Autodesk Inventor part; units mm, degrees
(part 2 of 3)
extrude "Extrusion14" add sketch "Sketch20" against normal blind 2.54 contours L123 L124 L125 L126 L127 L128 L129 L130 L131 L132 L133 L134 | L151 L152 L153 L154 L155 L156 | L181 L182 L183 L184 L185 L186 | L204 L197 L198 L199 L200 L201 L202 L203 | S194 S179 A0 | A0 S179 S180 S181 S182 S183 S184 L205 L206 S185 S186 S187 S188 S189 S190 S191 S192 L207 L208 S193 S194 | S73 S74 S75 S76 S77 S78 L135 L136 S79 S80 S81 S82 S83 S84 S85 S86 L137 L138 S87 S88 A0 | A0 S88 S73 | S92 S93 S94 S95 S96 S89 S90 S91 A0 | A0 S91 S92 | S167 S168 A0 | A0 S168 S169 S170 S171 S172 S165 S166 S167 | S153 S154 A0 | A0 S154 S155 S156 S157 S158 S151 S152 S153 | S103 L157 L158 S104 S105 S106 S107 S108 S109 S110 S111 L159 L160 S112 S113 S114 S115 S116 S117 S118 A0 | A0 S118 S103 | S150 S135 A0 | A0 S135 S136 S137 S138 S139 S140 L165 L166 S141 S142 S143 S144 S145 S146 S147 S148 L167 L168 S149 S150 | S119 L161 L162 S120 S121 S122 S123 S124 S125 S126 S127 L163 L164 S128 S129 S130 S131 S132 S133 S134 A0 | A0 S134 S119 | S0 S1 L0 L1 L2 L3 L4 S2 S3 | L8 L9 L10 L11 L12 L13 L14 L15 L16 L17 L18 L19 | L20 L21 L22 L23 L24 L25 L26 L27 L28 L29 L30 L31 | L32 L33 L34 L35 L36 L37 L38 S8 S9 S10 L39 | L43 L44 L45 L46 L47 L48 L49 L50 | L54 L55 L56 L57 L58 L59 L60 L61 L62 L63 L64 L65 L66 | L67 L68 L69 L70 L71 L72 L73 L74 | L78 L79 L80 L81 L82 L83 L84 S15 S16 S17 L85 | S22 S23 L89 L90 L91 S24 S25 | L95 L96 S30 S31 S32 S33 S34 S35 L97 L98 S36 S37 S38 S39 S40 L99 L100 | S41 S42 S43 S44 | L101 L102 L103 L104 L105 L106 S53 L107 L108 L109 L110 | S54 S55 S56 L111 S57 S58 S59 S60 L112 S61 S62 | L113 L114 L115 L116 L117 L118 L119 L120 L121 L122 | L139 L140 L141 L142 L143 L144 L145 L146 L147 L148 L149 L150 | L169 L170 L171 L172 L173 L174 L175 L176 L177 L178 L179 L180 | L187 L188 L189 L190 L191 L192 L193 L194 L195 L196
sketch "Sketch21" plane through (27.94, 0, 0) normal (1, 0, 0) x (0, 0, -1)
  point P0 (0, 0)
sketch "Sketch22" plane through (25.4, 0, 0) normal (1, 0, 0) x (0, 0, -1)
  circle A0 centre (0, 0) radius 75.606
  line L0 (-75.2037, 22.4511) -> (-75.7978, 19.48)
  line L1 (-75.7978, 19.48) -> (-94.7412, 14.099)
  line L2 (-94.7412, 14.099) -> (-77.5606, 10.6637)
  line L3 (-77.5606, 10.6637) -> (-78.0546, 8.1932)
  line L4 (-78.0546, 8.1932) -> (-97.9802, 12.1773)
  line L5 (-97.9802, 12.1773) -> (-97.2279, 15.9396)
  line L6 (-97.2279, 15.9396) -> (-79.8475, 20.8104)
  line L7 (-79.8475, 20.8104) -> (-95.6233, 23.9648)
  line L8 (-95.6233, 23.9648) -> (-95.1293, 26.4353)
  line L9 (-95.1293, 26.4353) -> (-75.2037, 22.4511)
  line L10 (-71.0246, 32.8287) -> (-73.9643, 25.5272)
  line L11 (-73.9643, 25.5272) -> (-75.8889, 26.3021)
  line L12 (-75.8889, 26.3021) -> (-74.9234, 28.7003)
  line L13 (-74.9234, 28.7003) -> (-89.9237, 34.7395)
  line L14 (-89.9237, 34.7395) -> (-90.8892, 32.3413)
  line L15 (-90.8892, 32.3413) -> (-92.8139, 33.1162)
  line L16 (-92.8139, 33.1162) -> (-89.8742, 40.4178)
  line L17 (-89.8742, 40.4178) -> (-87.9496, 39.6429)
  line L18 (-87.9496, 39.6429) -> (-88.9151, 37.2447)
  line L19 (-88.9151, 37.2447) -> (-73.9148, 31.2054)
  line L20 (-73.9148, 31.2054) -> (-72.9493, 33.6036)
  line L21 (-72.9493, 33.6036) -> (-71.0246, 32.8287)
  spline S0 degree 2 poles (-65.2074, 42.4368) (-66.2508, 40.7587) (-69.1486, 38.6243) (-70.9248, 38.2938) knots 0 0 0 1 2 2 2
  spline S1 degree 2 poles (-70.9248, 38.2938) (-72.6869, 37.9546) (-76.7474, 38.9088) (-78.9288, 40.2652) knots 0 0 0 1 2 2 2
  spline S2 degree 2 poles (-78.9288, 40.2652) (-81.0963, 41.613) (-83.6257, 44.7176) (-84.1622, 46.5055) knots 0 0 0 1 2 2 2
  spline S3 degree 2 poles (-84.1622, 46.5055) (-84.6794, 48.262) (-84.1396, 51.8432) (-83.0527, 53.5912) knots 0 0 0 1 2 2 2
  spline S4 degree 2 poles (-83.0527, 53.5912) (-82.5136, 54.4582) (-81.3141, 55.8259) (-80.7183, 56.3475) knots 0 0 0 1 2 2 2
  spline S5 degree 2 poles (-80.7183, 56.3475) (-80.1887, 56.7938) (-78.9496, 57.6327) (-78.2855, 58.0148) knots 0 0 0 1 2 2 2
  line L22 (-78.2855, 58.0148) -> (-75.5167, 56.2931)
  line L23 (-75.5167, 56.2931) -> (-75.6297, 56.1113)
  spline S6 degree 2 poles (-75.6297, 56.1113) (-76.1007, 55.9776) (-77.475, 55.5136) (-78.2787, 55.0632) knots 0 0 0 1 2 2 2
  spline S7 degree 2 poles (-78.2787, 55.0632) (-79.0509, 54.632) (-80.4776, 53.3667) (-81.1036, 52.3599) knots 0 0 0 1 2 2 2
  spline S8 degree 2 poles (-81.1036, 52.3599) (-81.7905, 51.2552) (-82.1076, 48.7183) (-81.7015, 47.438) knots 0 0 0 1 2 2 2
  spline S9 degree 2 poles (-81.7015, 47.438) (-81.2726, 46.1631) (-79.106, 43.6912) (-77.442, 42.6565) knots 0 0 0 1 2 2 2
  spline S10 degree 2 poles (-77.442, 42.6565) (-75.666, 41.5522) (-72.5766, 40.814) (-71.2347, 41.0073) knots 0 0 0 1 2 2 2
  spline S11 degree 2 poles (-71.2347, 41.0073) (-69.9296, 41.2041) (-67.8539, 42.6087) (-67.1757, 43.6995) knots 0 0 0 1 2 2 2
  spline S12 degree 2 poles (-67.1757, 43.6995) (-66.5583, 44.6923) (-65.9957, 46.6887) (-65.9506, 47.572) knots 0 0 0 1 2 2 2
  spline S13 degree 2 poles (-65.9506, 47.572) (-65.9229, 48.4274) (-66.0954, 49.8338) (-66.1959, 50.2647) knots 0 0 0 1 2 2 2
  line L24 (-66.1959, 50.2647) -> (-66.0916, 50.4325)
  line L25 (-66.0916, 50.4325) -> (-63.3507, 48.7283)
  spline S14 degree 2 poles (-63.3507, 48.7283) (-63.4415, 47.9897) (-63.5782, 46.6786) (-63.7979, 45.8263) knots 0 0 0 1 2 2 2
  spline S15 degree 2 poles (-63.7979, 45.8263) (-64.0157, 44.9146) (-64.5639, 43.4716) (-65.2074, 42.4368) knots 0 0 0 1 2 2 2
  line L26 (-50.1614, 60.3743) -> (-52.0671, 58.4609)
  line L27 (-52.0671, 58.4609) -> (-59.114, 65.4797)
  line L28 (-59.114, 65.4797) -> (-65.7144, 58.8529)
  line L29 (-65.7144, 58.8529) -> (-58.6676, 51.8341)
  line L30 (-58.6676, 51.8341) -> (-60.5734, 49.9207)
  line L31 (-60.5734, 49.9207) -> (-74.9704, 64.2605)
  line L32 (-74.9704, 64.2605) -> (-73.0646, 66.1739)
  line L33 (-73.0646, 66.1739) -> (-67.4178, 60.5495)
  line L34 (-67.4178, 60.5495) -> (-60.8173, 67.1763)
  line L35 (-60.8173, 67.1763) -> (-66.4641, 72.8007)
  line L36 (-66.4641, 72.8007) -> (-64.5583, 74.7141)
  line L37 (-64.5583, 74.7141) -> (-50.1614, 60.3743)
  spline S16 degree 2 poles (-43.9337, 85.7693) (-42.2501, 85.2061) (-39.1129, 82.481) (-37.8061, 80.3077) knots 0 0 0 1 2 2 2
  spline S17 degree 2 poles (-37.8061, 80.3077) (-36.5333, 78.1909) (-35.5439, 74.1168) (-35.8642, 72.3486) knots 0 0 0 1 2 2 2
  spline S18 degree 2 poles (-35.8642, 72.3486) (-36.2069, 70.4901) (-38.3477, 67.6273) (-40.0553, 66.6006) knots 0 0 0 1 2 2 2
  spline S19 degree 2 poles (-40.0553, 66.6006) (-41.8193, 65.5399) (-45.363, 65.0424) (-47.0974, 65.5943) knots 0 0 0 1 2 2 2
  spline S20 degree 2 poles (-47.0974, 65.5943) (-48.7952, 66.149) (-51.9127, 68.9052) (-53.2025, 71.0502) knots 0 0 0 1 2 2 2
  spline S21 degree 2 poles (-53.2025, 71.0502) (-54.5177, 73.2376) (-55.4336, 77.2214) (-55.1529, 79.0234) knots 0 0 0 1 2 2 2
  spline S22 degree 2 poles (-55.1529, 79.0234) (-54.8326, 80.7916) (-52.7174, 83.6967) (-50.9674, 84.7488) knots 0 0 0 1 2 2 2
  spline S23 degree 2 poles (-50.9674, 84.7488) (-49.1893, 85.818) (-45.5919, 86.2902) (-43.9337, 85.7693) knots 0 0 0 1 2 2 2
  spline S24 degree 2 poles (-40.2193, 78.8567) (-41.2545, 80.5784) (-43.6062, 82.7959) (-44.8097, 83.2636) knots 0 0 0 1 2 2 2
  spline S25 degree 2 poles (-44.8097, 83.2636) (-46.0442, 83.751) (-48.5348, 83.4831) (-49.7484, 82.7534) knots 0 0 0 1 2 2 2
  spline S26 degree 2 poles (-49.7484, 82.7534) (-51.0044, 81.9982) (-52.3693, 79.9862) (-52.529, 78.6221) knots 0 0 0 1 2 2 2
  spline S27 degree 2 poles (-52.529, 78.6221) (-52.6859, 77.3172) (-51.8075, 74.1947) (-50.7893, 72.5012) knots 0 0 0 1 2 2 2
  spline S28 degree 2 poles (-50.7893, 72.5012) (-48.7274, 69.0719) (-43.6593, 67.162) (-41.2461, 68.613) knots 0 0 0 1 2 2 2
  spline S29 degree 2 poles (-41.2461, 68.613) (-38.8329, 70.064) (-38.1573, 75.4275) (-40.2193, 78.8567) knots 0 0 0 1 2 2 2
  line L38 (-18.5674, 76.2196) -> (-29.718, 72.44)
  line L39 (-29.718, 72.44) -> (-36.2411, 91.6845)
  line L40 (-36.2411, 91.6845) -> (-33.6835, 92.5515)
  line L41 (-33.6835, 92.5515) -> (-27.9322, 75.5838)
  line L42 (-27.9322, 75.5838) -> (-19.3392, 78.4965)
  line L43 (-19.3392, 78.4965) -> (-18.5674, 76.2196)
  spline S30 degree 2 poles (-10.8247, 77.0268) (-13.01, 76.7214) (-16.2036, 77.2061) (-17.6484, 77.6692) knots 0 0 0 1 2 2 2
  line L44 (-17.6484, 77.6692) -> (-18.118, 81.0287)
  line L45 (-18.118, 81.0287) -> (-17.9223, 81.0561)
  spline S31 degree 2 poles (-17.9223, 81.0561) (-16.4281, 80.0013) (-12.8934, 79.0987) (-11.3441, 79.3153) knots 0 0 0 1 2 2 2
  spline S32 degree 2 poles (-11.3441, 79.3153) (-9.1262, 79.6253) (-7.1169, 81.785) (-7.3289, 83.3016) knots 0 0 0 1 2 2 2
  spline S33 degree 2 poles (-7.3289, 83.3016) (-7.4976, 84.5084) (-8.8978, 85.8424) (-10.2386, 86.0374) knots 0 0 0 1 2 2 2
  spline S34 degree 2 poles (-10.2386, 86.0374) (-11.2046, 86.1684) (-12.8041, 86.3106) (-14.003, 86.4423) knots 0 0 0 1 2 2 2
  spline S35 degree 2 poles (-14.003, 86.4423) (-15.0855, 86.5737) (-16.8489, 87.1752) (-17.5783, 87.7549) knots 0 0 0 1 2 2 2
  spline S36 degree 2 poles (-17.5783, 87.7549) (-18.2915, 88.3369) (-19.2272, 90.0351) (-19.3913, 91.2093) knots 0 0 0 1 2 2 2
  spline S37 degree 2 poles (-19.3913, 91.2093) (-19.7332, 93.6555) (-16.3799, 97.4995) (-13.4281, 97.9121) knots 0 0 0 1 2 2 2
  spline S38 degree 2 poles (-13.4281, 97.9121) (-11.732, 98.1492) (-8.6378, 97.8999) (-7.2606, 97.444) knots 0 0 0 1 2 2 2
  line L46 (-7.2606, 97.444) -> (-6.8138, 94.2476)
  line L47 (-6.8138, 94.2476) -> (-7.0095, 94.2202)
  spline S39 degree 2 poles (-7.0095, 94.2202) (-8.0948, 94.9664) (-11.2779, 95.8516) (-12.925, 95.6214) knots 0 0 0 1 2 2 2
  spline S40 degree 2 poles (-12.925, 95.6214) (-14.7841, 95.3615) (-16.8397, 93.2951) (-16.6414, 91.8763) knots 0 0 0 1 2 2 2
  spline S41 degree 2 poles (-16.6414, 91.8763) (-16.4636, 90.6043) (-14.898, 89.2768) (-13.5781, 89.1121) knots 0 0 0 1 2 2 2
  spline S42 degree 2 poles (-13.5781, 89.1121) (-12.6981, 89.0024) (-10.1535, 88.7595) (-9.3039, 88.6288) knots 0 0 0 1 2 2 2
  spline S43 degree 2 poles (-9.3039, 88.6288) (-7.1439, 88.2823) (-4.8616, 85.9909) (-4.5995, 84.1154) knots 0 0 0 1 2 2 2
  spline S44 degree 2 poles (-4.5995, 84.1154) (-4.4331, 82.9249) (-5.0761, 80.5073) (-5.8288, 79.5874) knots 0 0 0 1 2 2 2
  spline S45 degree 2 poles (-5.8288, 79.5874) (-6.6679, 78.5722) (-8.9819, 77.2844) (-10.8247, 77.0268) knots 0 0 0 1 2 2 2
  spline S46 degree 2 poles (13.192, 76.6569) (11.0177, 77.0327) (8.1242, 78.4687) (6.8896, 79.3505) knots 0 0 0 1 2 2 2
  line L48 (6.8896, 79.3505) -> (7.4674, 82.6931)
  line L49 (7.4674, 82.6931) -> (7.6621, 82.6595)
  spline S47 degree 2 poles (7.6621, 82.6595) (8.7633, 81.1991) (11.854, 79.2611) (13.3955, 78.9947) knots 0 0 0 1 2 2 2
  spline S48 degree 2 poles (13.3955, 78.9947) (15.6023, 78.6132) (18.1747, 80.0569) (18.4355, 81.566) knots 0 0 0 1 2 2 2
  spline S49 degree 2 poles (18.4355, 81.566) (18.6431, 82.7667) (17.7166, 84.4642) (16.4992, 85.059) knots 0 0 0 1 2 2 2
  spline S50 degree 2 poles (16.4992, 85.059) (15.6192, 85.4785) (14.1394, 86.1019) (13.0379, 86.5932) knots 0 0 0 1 2 2 2
  spline S51 degree 2 poles (13.0379, 86.5932) (12.0471, 87.0485) (10.5513, 88.1593) (10.0334, 88.934) knots 0 0 0 1 2 2 2
  spline S52 degree 2 poles (10.0334, 88.934) (9.5318, 89.7058) (9.1589, 91.6085) (9.3608, 92.7768) knots 0 0 0 1 2 2 2
  spline S53 degree 2 poles (9.3608, 92.7768) (9.7815, 95.2107) (14.1478, 97.8483) (17.0847, 97.3406) knots 0 0 0 1 2 2 2
  spline S54 degree 2 poles (17.0847, 97.3406) (18.7723, 97.0489) (21.6429, 95.8676) (22.8154, 95.0132) knots 0 0 0 1 2 2 2
  line L50 (22.8154, 95.0132) -> (22.2656, 91.8329)
  line L51 (22.2656, 91.8329) -> (22.0709, 91.8665)
  spline S55 degree 2 poles (22.0709, 91.8665) (21.265, 92.9082) (18.5038, 94.7224) (16.865, 95.0057) knots 0 0 0 1 2 2 2
  spline S56 degree 2 poles (16.865, 95.0057) (15.0152, 95.3254) (12.4272, 93.9847) (12.1832, 92.573) knots 0 0 0 1 2 2 2
  spline S57 degree 2 poles (12.1832, 92.573) (11.9644, 91.3074) (13.0503, 89.5656) (14.2571, 89.006) knots 0 0 0 1 2 2 2
  spline S58 degree 2 poles (14.2571, 89.006) (15.0616, 88.633) (17.4107, 87.6254) (18.18, 87.2417) knots 0 0 0 1 2 2 2
  spline S59 degree 2 poles (18.18, 87.2417) (20.1313, 86.2527) (21.6056, 83.3742) (21.2831, 81.5082) knots 0 0 0 1 2 2 2
  spline S60 degree 2 poles (21.2831, 81.5082) (21.0784, 80.3237) (19.7283, 78.2175) (18.7309, 77.5711) knots 0 0 0 1 2 2 2
  spline S61 degree 2 poles (18.7309, 77.5711) (17.6221, 76.8604) (15.0255, 76.34) (13.192, 76.6569) knots 0 0 0 1 2 2 2
  spline S62 degree 2 poles (30.1527, 71.7196) (28.3157, 72.4477) (25.6996, 74.9193) (25.0582, 76.6083) knots 0 0 0 1 2 2 2
  spline S63 degree 2 poles (25.0582, 76.6083) (24.4108, 78.2819) (24.627, 82.4473) (25.5735, 84.8354) knots 0 0 0 1 2 2 2
  spline S64 degree 2 poles (25.5735, 84.8354) (26.5139, 87.2082) (29.1188, 90.2498) (30.7826, 91.0959) knots 0 0 0 1 2 2 2
  spline S65 degree 2 poles (30.7826, 91.0959) (32.419, 91.9175) (36.0391, 92.0237) (37.9527, 91.2653) knots 0 0 0 1 2 2 2
  spline S66 degree 2 poles (37.9527, 91.2653) (38.9018, 90.8891) (40.4612, 89.9523) (41.0804, 89.4588) knots 0 0 0 1 2 2 2
  spline S67 degree 2 poles (41.0804, 89.4588) (41.6139, 89.0171) (42.66, 87.9471) (43.1541, 87.3616) knots 0 0 0 1 2 2 2
  line L52 (43.1541, 87.3616) -> (41.9528, 84.3306)
  line L53 (41.9528, 84.3306) -> (41.7538, 84.4094)
  spline S68 degree 2 poles (41.7538, 84.4094) (41.5383, 84.8491) (40.8371, 86.1189) (40.2509, 86.8296) knots 0 0 0 1 2 2 2
  spline S69 degree 2 poles (40.2509, 86.8296) (39.6891, 87.5127) (38.1901, 88.6914) (37.0879, 89.1282) knots 0 0 0 1 2 2 2
  spline S70 degree 2 poles (37.0879, 89.1282) (35.8786, 89.6075) (33.3257, 89.468) (32.1382, 88.8405) knots 0 0 0 1 2 2 2
  spline S71 degree 2 poles (32.1382, 88.8405) (30.96, 88.1915) (28.9132, 85.6196) (28.1912, 83.7979) knots 0 0 0 1 2 2 2
  spline S72 degree 2 poles (28.1912, 83.7979) (27.4207, 81.8538) (27.2441, 78.6822) (27.6732, 77.3963) knots 0 0 0 1 2 2 2
  spline S73 degree 2 poles (27.6732, 77.3963) (28.0992, 76.1469) (29.8508, 74.3545) (31.0449, 73.8812) knots 0 0 0 1 2 2 2
  spline S74 degree 2 poles (31.0449, 73.8812) (32.1318, 73.4504) (34.1964, 73.2521) (35.0736, 73.3649) knots 0 0 0 1 2 2 2
  spline S75 degree 2 poles (35.0736, 73.3649) (35.9203, 73.4899) (37.2736, 73.9101) (37.6797, 74.0856) knots 0 0 0 1 2 2 2
  line L54 (37.6797, 74.0856) -> (37.8634, 74.0128)
  line L55 (37.8634, 74.0128) -> (36.6742, 71.0124)
  spline S76 degree 2 poles (36.6742, 71.0124) (35.9313, 70.9703) (34.6167, 70.8714) (33.7389, 70.9359) knots 0 0 0 1 2 2 2
  spline S77 degree 2 poles (33.7389, 70.9359) (32.8031, 70.988) (31.2855, 71.2706) (30.1527, 71.7196) knots 0 0 0 1 2 2 2
  line L56 (50.4819, 60.1066) -> (48.2598, 61.6413)
  line L57 (48.2598, 61.6413) -> (53.9123, 69.8249)
  line L58 (53.9123, 69.8249) -> (46.2165, 75.1405)
  line L59 (46.2165, 75.1405) -> (40.564, 66.9569)
  line L60 (40.564, 66.9569) -> (38.342, 68.4917)
  line L61 (38.342, 68.4917) -> (49.8902, 85.2111)
  line L62 (49.8902, 85.2111) -> (52.1122, 83.6764)
  line L63 (52.1122, 83.6764) -> (47.5828, 77.1187)
  line L64 (47.5828, 77.1187) -> (55.2786, 71.8031)
  line L65 (55.2786, 71.8031) -> (59.8081, 78.3608)
  line L66 (59.8081, 78.3608) -> (62.0301, 76.826)
  line L67 (62.0301, 76.826) -> (50.4819, 60.1066)
  spline S78 degree 2 poles (76.5798, 58.4985) (76.3253, 56.7415) (74.2021, 53.1693) (72.2961, 51.4966) knots 0 0 0 1 2 2 2
  spline S79 degree 2 poles (72.2961, 51.4966) (70.4397, 49.8674) (66.6067, 48.1686) (64.8098, 48.169) knots 0 0 0 1 2 2 2
  spline S80 degree 2 poles (64.8098, 48.169) (62.9199, 48.1755) (59.7218, 49.7725) (58.4076, 51.2701) knots 0 0 0 1 2 2 2
  spline S81 degree 2 poles (58.4076, 51.2701) (57.0498, 52.8171) (55.9295, 56.2157) (56.1638, 58.0207) knots 0 0 0 1 2 2 2
  spline S82 degree 2 poles (56.1638, 58.0207) (56.4075, 59.7901) (58.5648, 63.3484) (60.446, 64.9994) knots 0 0 0 1 2 2 2
  spline S83 degree 2 poles (60.446, 64.9994) (62.3643, 66.6829) (66.1216, 68.2933) (67.9447, 68.3378) knots 0 0 0 1 2 2 2
  spline S84 degree 2 poles (67.9447, 68.3378) (69.7417, 68.3374) (72.9769, 66.773) (74.3237, 65.2383) knots 0 0 0 1 2 2 2
  spline S85 degree 2 poles (74.3237, 65.2383) (75.6923, 63.6788) (76.7972, 60.223) (76.5798, 58.4985) knots 0 0 0 1 2 2 2
  spline S86 degree 2 poles (70.4388, 53.613) (71.9487, 54.9381) (73.7122, 57.647) (73.9582, 58.9145) knots 0 0 0 1 2 2 2
  spline S87 degree 2 poles (73.9582, 58.9145) (74.2181, 60.216) (73.5112, 62.6192) (72.5771, 63.6835) knots 0 0 0 1 2 2 2
  spline S88 degree 2 poles (72.5771, 63.6835) (71.6104, 64.785) (69.3876, 65.7701) (68.0168, 65.6844) knots 0 0 0 1 2 2 2
  spline S89 degree 2 poles (68.0168, 65.6844) (66.7049, 65.6065) (63.7885, 64.1864) (62.3033, 62.883) knots 0 0 0 1 2 2 2
  spline S90 degree 2 poles (62.3033, 62.883) (59.2959, 60.2436) (58.3185, 54.9164) (60.1759, 52.8001) knots 0 0 0 1 2 2 2
  spline S91 degree 2 poles (60.1759, 52.8001) (62.0332, 50.6837) (67.4313, 50.9736) (70.4388, 53.613) knots 0 0 0 1 2 2 2
  spline S92 degree 2 poles (88.7372, 37.5799) (88.0531, 35.9417) (85.1071, 33.0109) (82.8445, 31.8657) knots 0 0 0 1 2 2 2
  spline S93 degree 2 poles (82.8445, 31.8657) (80.6407, 30.7502) (76.5054, 30.0597) (74.7652, 30.5077) knots 0 0 0 1 2 2 2
  spline S94 degree 2 poles (74.7652, 30.5077) (72.9366, 30.9848) (70.2371, 33.328) (69.3372, 35.1057) knots 0 0 0 1 2 2 2
  spline S95 degree 2 poles (69.3372, 35.1057) (68.4077, 36.9422) (68.1691, 40.5127) (68.8457, 42.2025) knots 0 0 0 1 2 2 2
  spline S96 degree 2 poles (68.8457, 42.2025) (69.5224, 43.8554) (72.498, 46.7642) (74.7312, 47.8946) knots 0 0 0 1 2 2 2
  spline S97 degree 2 poles (74.7312, 47.8946) (77.0084, 49.0472) (81.0483, 49.671) (82.8251, 49.26) knots 0 0 0 1 2 2 2
  spline S98 degree 2 poles (82.8251, 49.26) (84.5653, 48.812) (87.3089, 46.491) (88.231, 44.6692) knots 0 0 0 1 2 2 2
  spline S99 degree 2 poles (88.231, 44.6692) (89.168, 42.818) (89.3773, 39.1959) (88.7372, 37.5799) knots 0 0 0 1 2 2 2
  spline S100 degree 2 poles (81.5728, 34.378) (83.3653, 35.2853) (85.7479, 37.4695) (86.3018, 38.6358) knots 0 0 0 1 2 2 2
  spline S101 degree 2 poles (86.3018, 38.6358) (86.8777, 39.8316) (86.7917, 42.335) (86.1522, 43.5985) knots 0 0 0 1 2 2 2
  spline S102 degree 2 poles (86.1522, 43.5985) (85.4903, 44.9061) (83.5829, 46.4137) (82.234, 46.6722) knots 0 0 0 1 2 2 2
  spline S103 degree 2 poles (82.234, 46.6722) (80.944, 46.9236) (77.7658, 46.2746) (76.0028, 45.3822) knots 0 0 0 1 2 2 2
  spline S104 degree 2 poles (76.0028, 45.3822) (72.4327, 43.5751) (70.1593, 38.6594) (71.4309, 36.147) knots 0 0 0 1 2 2 2
  spline S105 degree 2 poles (71.4309, 36.147) (72.7026, 33.6347) (78.0027, 32.5709) (81.5728, 34.378) knots 0 0 0 1 2 2 2
  line L68 (77.3681, 12.9753) -> (74.4094, 24.3712)
  line L69 (74.4094, 24.3712) -> (94.0774, 29.4775)
  line L70 (94.0774, 29.4775) -> (94.756, 26.8636)
  line L71 (94.756, 26.8636) -> (77.415, 22.3614)
  line L72 (77.415, 22.3614) -> (79.6951, 13.5794)
  line L73 (79.6951, 13.5794) -> (77.3681, 12.9753)
  line L74 (95.7165, -10.6849) -> (96.0871, -1.2402)
  line L75 (96.0871, -1.2402) -> (90.3611, -1.0156)
  line L76 (90.3611, -1.0156) -> (90.006, -10.0653)
  line L77 (90.006, -10.0653) -> (87.6037, -9.9711)
  line L78 (87.6037, -9.9711) -> (87.9588, -0.9213)
  line L79 (87.9588, -0.9213) -> (78.185, -0.5379)
  line L80 (78.185, -0.5379) -> (78.2909, 2.1606)
  line L81 (78.2909, 2.1606) -> (98.5953, 1.364)
  line L82 (98.5953, 1.364) -> (98.1188, -10.7791)
  line L83 (98.1188, -10.7791) -> (95.7165, -10.6849)
  line L84 (73.6659, -27.626) -> (74.5088, -24.2214)
  line L85 (74.5088, -24.2214) -> (83.9003, -19.9304)
  line L86 (83.9003, -19.9304) -> (84.6442, -16.9254)
  line L87 (84.6442, -16.9254) -> (76.7959, -14.9825)
  line L88 (76.7959, -14.9825) -> (77.4449, -12.3611)
  line L89 (77.4449, -12.3611) -> (97.1695, -17.244)
  line L90 (97.1695, -17.244) -> (95.9111, -22.327)
  spline S106 degree 2 poles (95.9111, -22.327) (95.4917, -24.0214) (94.5582, -26.2161) (93.6297, -27.0889) knots 0 0 0 1 2 2 2
  spline S107 degree 2 poles (93.6297, -27.0889) (92.7011, -27.9617) (90.3104, -28.6421) (88.7599, -28.2583) knots 0 0 0 1 2 2 2
  spline S108 degree 2 poles (88.7599, -28.2583) (86.602, -27.7241) (84.223, -24.7941) (83.9866, -22.7339) knots 0 0 0 1 2 2 2
  line L91 (83.9866, -22.7339) -> (73.6659, -27.626)
  spline S109 degree 2 poles (89.2288, -25.4735) (90.0919, -25.6872) (91.569, -25.4082) (92.1588, -24.8757) knots 0 0 0 1 2 2 2
  spline S110 degree 2 poles (92.1588, -24.8757) (92.665, -24.4073) (93.3367, -22.9959) (93.6058, -21.909) knots 0 0 0 1 2 2 2
  line L92 (93.6058, -21.909) -> (94.2507, -19.3035)
  line L93 (94.2507, -19.3035) -> (86.8341, -17.4675)
  line L94 (86.8341, -17.4675) -> (86.2642, -19.7692)
  spline S111 degree 2 poles (86.2642, -19.7692) (85.9833, -20.9041) (85.9358, -22.8093) (86.4048, -23.587) knots 0 0 0 1 2 2 2
  spline S112 degree 2 poles (86.4048, -23.587) (86.8058, -24.2969) (88.2058, -25.2203) (89.2288, -25.4735) knots 0 0 0 1 2 2 2
  spline S113 degree 2 poles (68.9812, -35.9789) (69.8586, -34.2084) (72.5381, -31.8056) (74.2743, -31.306) knots 0 0 0 1 2 2 2
  spline S114 degree 2 poles (74.2743, -31.306) (75.9957, -30.7992) (80.129, -31.359) (82.4307, -32.4997) knots 0 0 0 1 2 2 2
  spline S115 degree 2 poles (82.4307, -32.4997) (84.7176, -33.6331) (87.5334, -36.4805) (88.2391, -38.2086) knots 0 0 0 1 2 2 2
  spline S116 degree 2 poles (88.2391, -38.2086) (88.9226, -39.9073) (88.7292, -43.5238) (87.8151, -45.3681) knots 0 0 0 1 2 2 2
  spline S117 degree 2 poles (87.8151, -45.3681) (87.3618, -46.2829) (86.2992, -47.7595) (85.7563, -48.3358) knots 0 0 0 1 2 2 2
  spline S118 degree 2 poles (85.7563, -48.3358) (85.272, -48.8309) (84.1191, -49.7849) (83.4948, -50.229) knots 0 0 0 1 2 2 2
  line L95 (83.4948, -50.229) -> (80.5734, -48.7812)
  line L96 (80.5734, -48.7812) -> (80.6685, -48.5894)
  spline S119 degree 2 poles (80.6685, -48.5894) (81.1244, -48.411) (82.4479, -47.8172) (83.2046, -47.2917) knots 0 0 0 1 2 2 2
  spline S120 degree 2 poles (83.2046, -47.2917) (83.9318, -46.7884) (85.2304, -45.392) (85.7569, -44.3297) knots 0 0 0 1 2 2 2
  spline S121 degree 2 poles (85.7569, -44.3297) (86.3345, -43.1641) (86.4065, -40.6084) (85.8793, -39.3731) knots 0 0 0 1 2 2 2
  spline S122 degree 2 poles (85.8793, -39.3731) (85.33, -38.1452) (82.9361, -35.8929) (81.1803, -35.0227) knots 0 0 0 1 2 2 2
  spline S123 degree 2 poles (81.1803, -35.0227) (79.3065, -34.0941) (76.1605, -33.6559) (74.8434, -33.9772) knots 0 0 0 1 2 2 2
  spline S124 degree 2 poles (74.8434, -33.9772) (73.5632, -34.2984) (71.632, -35.8959) (71.0617, -37.0467) knots 0 0 0 1 2 2 2
  spline S125 degree 2 poles (71.0617, -37.0467) (70.5425, -38.0943) (70.1741, -40.1355) (70.2141, -41.019) knots 0 0 0 1 2 2 2
  spline S126 degree 2 poles (70.2141, -41.019) (70.2686, -41.8731) (70.5754, -43.2565) (70.7168, -43.6757) knots 0 0 0 1 2 2 2
  line L97 (70.7168, -43.6757) -> (70.6291, -43.8528)
  line L98 (70.6291, -43.8528) -> (67.7373, -42.4196)
  spline S127 degree 2 poles (67.7373, -42.4196) (67.7567, -41.6757) (67.7668, -40.3575) (67.9037, -39.4881) knots 0 0 0 1 2 2 2
  spline S128 degree 2 poles (67.9037, -39.4881) (68.0329, -38.5597) (68.4401, -37.0707) (68.9812, -35.9789) knots 0 0 0 1 2 2 2
  spline S129 degree 2 poles (-82.6802, -17.8177) (-83.9869, -17.9846) (-86.458, -17.3541) (-87.3811, -16.6254) knots 0 0 0 1 2 2 2
  spline S130 degree 2 poles (-87.3811, -16.6254) (-88.5437, -15.7115) (-89.9665, -13.0214) (-90.2419, -10.8653) knots 0 0 0 1 2 2 2
  line L99 (-90.2419, -10.8653) -> (-90.532, -8.5948)
  line L100 (-90.532, -8.5948) -> (-98.0456, -9.5548)
  line L101 (-98.0456, -9.5548) -> (-98.3879, -6.876)
  line L102 (-98.3879, -6.876) -> (-78.2317, -4.3009)
  line L103 (-78.2317, -4.3009) -> (-77.5848, -9.3644)
  spline S131 degree 2 poles (-77.5848, -9.3644) (-77.3552, -11.1611) (-77.6219, -13.7517) (-78.1685, -14.801) knots 0 0 0 1 2 2 2
  spline S132 degree 2 poles (-78.1685, -14.801) (-78.7922, -16.0261) (-80.9978, -17.6027) (-82.6802, -17.8177) knots 0 0 0 1 2 2 2
  spline S133 degree 2 poles (-83.1187, -15.035) (-82.0734, -14.9014) (-80.6298, -13.9866) (-80.2337, -13.1889) knots 0 0 0 1 2 2 2
  spline S134 degree 2 poles (-80.2337, -13.1889) (-79.8904, -12.4977) (-79.7644, -10.7551) (-79.9251, -9.4974) knots 0 0 0 1 2 2 2
  line L104 (-79.9251, -9.4974) -> (-80.2089, -7.276)
  line L105 (-80.2089, -7.276) -> (-88.2452, -8.3027)
  line L106 (-88.2452, -8.3027) -> (-88.0115, -10.1321)
  spline S135 degree 2 poles (-88.0115, -10.1321) (-87.8028, -11.7655) (-87.0234, -13.7078) (-86.2539, -14.2735) knots 0 0 0 1 2 2 2
  spline S136 degree 2 poles (-86.2539, -14.2735) (-85.5724, -14.8007) (-84.0824, -15.1581) (-83.1187, -15.035) knots 0 0 0 1 2 2 2
  line L107 (-96.1276, -22.1005) -> (-76.6251, -16.395)
  line L108 (-76.6251, -16.395) -> (-73.0557, -28.5959)
  line L109 (-73.0557, -28.5959) -> (-75.3631, -29.271)
  line L110 (-75.3631, -29.271) -> (-78.1743, -19.6619)
  line L111 (-78.1743, -19.6619) -> (-83.5161, -21.2247)
  line L112 (-83.5161, -21.2247) -> (-80.8945, -30.1858)
  line L113 (-80.8945, -30.1858) -> (-83.202, -30.8608)
  line L114 (-83.202, -30.8608) -> (-85.8236, -21.8998)
  line L115 (-85.8236, -21.8998) -> (-93.0619, -24.0174)
  line L116 (-93.0619, -24.0174) -> (-90.2508, -33.6264)
  line L117 (-90.2508, -33.6264) -> (-92.5582, -34.3015)
  line L118 (-92.5582, -34.3015) -> (-96.1276, -22.1005)
  line L119 (-91.4207, -37.0299) -> (-73.0664, -28.3109)
  line L120 (-73.0664, -28.3109) -> (-67.6117, -39.7934)
  line L121 (-67.6117, -39.7934) -> (-69.7832, -40.825)
  line L122 (-69.7832, -40.825) -> (-74.0792, -31.7818)
  line L123 (-74.0792, -31.7818) -> (-79.1065, -34.17)
  line L124 (-79.1065, -34.17) -> (-75.1003, -42.6034)
  line L125 (-75.1003, -42.6034) -> (-77.2719, -43.635)
  line L126 (-77.2719, -43.635) -> (-81.2781, -35.2016)
  line L127 (-81.2781, -35.2016) -> (-88.0903, -38.4376)
  line L128 (-88.0903, -38.4376) -> (-83.7944, -47.4809)
  line L129 (-83.7944, -47.4809) -> (-85.966, -48.5125)
  line L130 (-85.966, -48.5125) -> (-91.4207, -37.0299)
  line L131 (-75.4388, -63.9344) -> (-77.4502, -61.0611)
  line L132 (-77.4502, -61.0611) -> (-74.5095, -51.1633)
  line L133 (-74.5095, -51.1633) -> (-76.2848, -48.6272)
  line L134 (-76.2848, -48.6272) -> (-82.9084, -53.2639)
  line L135 (-82.9084, -53.2639) -> (-84.4571, -51.0515)
  line L136 (-84.4571, -51.0515) -> (-67.8105, -39.3985)
  line L137 (-67.8105, -39.3985) -> (-64.8075, -43.6883)
  spline S137 degree 2 poles (-64.8075, -43.6883) (-63.8065, -45.1183) (-62.7664, -47.2645) (-62.7192, -48.538) knots 0 0 0 1 2 2 2
  spline S138 degree 2 poles (-62.7192, -48.538) (-62.672, -49.8115) (-63.7309, -52.0603) (-65.0394, -52.9763) knots 0 0 0 1 2 2 2
  spline S139 degree 2 poles (-65.0394, -52.9763) (-66.8606, -54.2511) (-70.6324, -54.1176) (-72.3403, -52.9413) knots 0 0 0 1 2 2 2
  line L138 (-72.3403, -52.9413) -> (-75.4388, -63.9344)
  spline S140 degree 2 poles (-66.8296, -50.7922) (-66.1011, -50.2823) (-65.3403, -48.9859) (-65.3538, -48.1913) knots 0 0 0 1 2 2 2
  spline S141 degree 2 poles (-65.3538, -48.1913) (-65.3741, -47.502) (-65.996, -46.068) (-66.6381, -45.1507) knots 0 0 0 1 2 2 2
  line L139 (-66.6381, -45.1507) -> (-68.1774, -42.9518)
  line L140 (-68.1774, -42.9518) -> (-74.4367, -47.3335)
  line L141 (-74.4367, -47.3335) -> (-73.0769, -49.276)
  spline S142 degree 2 poles (-73.0769, -49.276) (-72.4064, -50.2338) (-71.0021, -51.5221) (-70.1077, -51.6799) knots 0 0 0 1 2 2 2
  spline S143 degree 2 poles (-70.1077, -51.6799) (-69.3091, -51.8445) (-67.693, -51.3966) (-66.8296, -50.7922) knots 0 0 0 1 2 2 2
  line L142 (-69.865, -69.9226) -> (-51.564, -58.7466)
  line L143 (-51.564, -58.7466) -> (-49.0144, -60.8829)
  line L144 (-49.0144, -60.8829) -> (-56.814, -80.8578)
  line L145 (-56.814, -80.8578) -> (-58.9975, -79.0282)
  line L146 (-58.9975, -79.0282) -> (-56.7626, -73.4892)
  line L147 (-56.7626, -73.4892) -> (-62.7075, -68.5081)
  line L148 (-62.7075, -68.5081) -> (-67.7697, -71.6782)
  line L149 (-67.7697, -71.6782) -> (-69.865, -69.9226)
  line L150 (-55.85, -71.2462) -> (-52.1164, -61.893)
  line L151 (-52.1164, -61.893) -> (-60.659, -67.2169)
  line L152 (-60.659, -67.2169) -> (-55.85, -71.2462)
  line L153 (-25.5281, -74.8652) -> (-39.5007, -90.477)
  line L154 (-39.5007, -90.477) -> (-42.1826, -89.0673)
  line L155 (-42.1826, -89.0673) -> (-37.9961, -72.2185)
  line L156 (-37.9961, -72.2185) -> (-49.3978, -85.275)
  line L157 (-49.3978, -85.275) -> (-52.0506, -83.8806)
  line L158 (-52.0506, -83.8806) -> (-47.188, -63.4805)
  line L159 (-47.188, -63.4805) -> (-44.7246, -64.7753)
  line L160 (-44.7246, -64.7753) -> (-48.9473, -81.5865)
  line L161 (-48.9473, -81.5865) -> (-37.5241, -68.56)
  line L162 (-37.5241, -68.56) -> (-35.0899, -69.8394)
  line L163 (-35.0899, -69.8394) -> (-39.4045, -86.8256)
  line L164 (-39.4045, -86.8256) -> (-27.8748, -73.6318)
  line L165 (-27.8748, -73.6318) -> (-25.5281, -74.8652)
  line L166 (-34.6364, -92.5776) -> (-22.6067, -74.8262)
  line L167 (-22.6067, -74.8262) -> (-19.4013, -75.7148)
  line L168 (-19.4013, -75.7148) -> (-18.2286, -97.1263)
  line L169 (-18.2286, -97.1263) -> (-20.9739, -96.3652)
  line L170 (-20.9739, -96.3652) -> (-21.2334, -90.398)
  line L171 (-21.2334, -90.398) -> (-28.7073, -88.326)
  line L172 (-28.7073, -88.326) -> (-32.0023, -93.3078)
  line L173 (-32.0023, -93.3078) -> (-34.6364, -92.5776)
  line L174 (-21.3316, -87.9785) -> (-21.8065, -77.9188)
  line L175 (-21.8065, -77.9188) -> (-27.3774, -86.3024)
  line L176 (-27.3774, -86.3024) -> (-21.3316, -87.9785)
  line L177 (-0.4026, -98.8861) -> (-3.8937, -98.5486)
  line L178 (-3.8937, -98.5486) -> (-9.508, -89.883)
  line L179 (-9.508, -89.883) -> (-12.5894, -89.5851)
  line L180 (-12.5894, -89.5851) -> (-13.3674, -97.6328)
  line L181 (-13.3674, -97.6328) -> (-16.0554, -97.3729)
  line L182 (-16.0554, -97.3729) -> (-14.1001, -77.1472)
  line L183 (-14.1001, -77.1472) -> (-8.888, -77.6511)
  spline S144 degree 2 poles (-8.888, -77.6511) (-7.1506, -77.819) (-4.8433, -78.4226) (-3.8444, -79.214) knots 0 0 0 1 2 2 2
  spline S145 degree 2 poles (-3.8444, -79.214) (-2.8456, -80.0054) (-1.8239, -82.2713) (-1.9776, -83.8612) knots 0 0 0 1 2 2 2
  spline S146 degree 2 poles (-1.9776, -83.8612) (-2.1915, -86.0739) (-4.7433, -88.8547) (-6.7471, -89.3889) knots 0 0 0 1 2 2 2
  line L184 (-6.7471, -89.3889) -> (-0.4026, -98.8861)
  spline S147 degree 2 poles (-4.8009, -83.8033) (-4.7154, -82.9182) (-5.2067, -81.4976) (-5.8195, -80.9917) knots 0 0 0 1 2 2 2
  spline S148 degree 2 poles (-5.8195, -80.9917) (-6.3568, -80.5593) (-7.8509, -80.1005) (-8.9655, -79.9928) knots 0 0 0 1 2 2 2
  line L185 (-8.9655, -79.9928) -> (-11.6371, -79.7345)
  line L186 (-11.6371, -79.7345) -> (-12.3723, -87.3396)
  line L187 (-12.3723, -87.3396) -> (-10.0121, -87.5678)
  spline S149 degree 2 poles (-10.0121, -87.5678) (-8.8484, -87.6803) (-6.9567, -87.4496) (-6.2557, -86.8721) knots 0 0 0 1 2 2 2
  spline S150 degree 2 poles (-6.2557, -86.8721) (-5.6117, -86.3719) (-4.9023, -84.8523) (-4.8009, -83.8033) knots 0 0 0 1 2 2 2
  spline S151 degree 2 poles (16.2804, -87.2344) (16.5233, -90.0066) (14.6669, -94.6654) (12.8897, -96.0774) knots 0 0 0 1 2 2 2
  spline S152 degree 2 poles (12.8897, -96.0774) (11.4325, -97.1803) (8.324, -98.1139) (5.8634, -98.3295) knots 0 0 0 1 2 2 2
  line L188 (5.8634, -98.3295) -> (1.2047, -98.7377)
  line L189 (1.2047, -98.7377) -> (-0.5689, -78.4952)
  line L190 (-0.5689, -78.4952) -> (4.0406, -78.0914)
  spline S153 degree 2 poles (4.0406, -78.0914) (6.8949, -77.8413) (10.2176, -78.4097) (11.432, -79.0636) knots 0 0 0 1 2 2 2
  spline S154 degree 2 poles (11.432, -79.0636) (13.4976, -80.1885) (16.0216, -84.2816) (16.2804, -87.2344) knots 0 0 0 1 2 2 2
  spline S155 degree 2 poles (13.4724, -87.4473) (13.2683, -85.118) (11.4374, -81.9559) (9.83, -81.1545) knots 0 0 0 1 2 2 2
  spline S156 degree 2 poles (9.83, -81.1545) (8.6912, -80.6096) (6.1967, -80.2497) (4.3759, -80.4092) knots 0 0 0 1 2 2 2
  line L191 (4.3759, -80.4092) -> (2.3254, -80.5889)
  line L192 (2.3254, -80.5889) -> (3.6909, -96.1726)
  line L193 (3.6909, -96.1726) -> (5.7414, -95.9929)
  spline S157 degree 2 poles (5.7414, -95.9929) (7.5294, -95.8363) (10.1857, -95.025) (11.2172, -94.1577) knots 0 0 0 1 2 2 2
  spline S158 degree 2 poles (11.2172, -94.1577) (12.5446, -93.0827) (13.6794, -89.8095) (13.4724, -87.4473) knots 0 0 0 1 2 2 2
  line L194 (39.6928, -90.3374) -> (27.9178, -94.6249)
  line L195 (27.9178, -94.6249) -> (26.9319, -91.9171)
  spline S159 degree 2 poles (26.9319, -91.9171) (27.7669, -90.2637) (29.2203, -87.2285) (29.8696, -85.6427) knots 0 0 0 1 2 2 2
  spline S160 degree 2 poles (29.8696, -85.6427) (31.178, -82.45) (31.7238, -78.9917) (31.166, -77.4599) knots 0 0 0 1 2 2 2
  spline S161 degree 2 poles (31.166, -77.4599) (30.8731, -76.6553) (29.9385, -75.6287) (29.3489, -75.4053) knots 0 0 0 1 2 2 2
  spline S162 degree 2 poles (29.3489, -75.4053) (28.7593, -75.1818) (27.4426, -75.2232) (26.7308, -75.4824) knots 0 0 0 1 2 2 2
  spline S163 degree 2 poles (26.7308, -75.4824) (26.05, -75.7303) (24.7814, -76.5777) (24.2427, -77.0718) knots 0 0 0 1 2 2 2
  spline S164 degree 2 poles (24.2427, -77.0718) (23.7801, -77.4856) (22.9997, -78.4707) (22.7691, -78.8) knots 0 0 0 1 2 2 2
  line L196 (22.7691, -78.8) -> (22.6298, -78.8507)
  line L197 (22.6298, -78.8507) -> (21.6383, -76.1275)
  spline S165 degree 2 poles (21.6383, -76.1275) (22.2865, -75.4533) (24.842, -73.6641) (26.1108, -73.2021) knots 0 0 0 1 2 2 2
  spline S166 degree 2 poles (26.1108, -73.2021) (28.7876, -72.2274) (32.8359, -73.9604) (33.7148, -76.3742) knots 0 0 0 1 2 2 2
  spline S167 degree 2 poles (33.7148, -76.3742) (34.1261, -77.5037) (34.2873, -79.5829) (34.1161, -80.5566) knots 0 0 0 1 2 2 2
  spline S168 degree 2 poles (34.1161, -80.5566) (33.9561, -81.5611) (33.2072, -83.6914) (32.7518, -84.751) knots 0 0 0 1 2 2 2
  spline S169 degree 2 poles (32.7518, -84.751) (32.0238, -86.5056) (30.0939, -90.3978) (29.5105, -91.539) knots 0 0 0 1 2 2 2
  line L198 (29.5105, -91.539) -> (38.8871, -88.1248)
  line L199 (38.8871, -88.1248) -> (39.6928, -90.3374)
  spline S170 degree 2 poles (48.3224, -74.197) (50.9614, -78.9849) (50.6501, -85.004) (47.7514, -86.6017) knots 0 0 0 1 2 2 2
  spline S171 degree 2 poles (47.7514, -86.6017) (44.8095, -88.2232) (39.5353, -85.1698) (36.952, -80.4829) knots 0 0 0 1 2 2 2
  spline S172 degree 2 poles (36.952, -80.4829) (34.2971, -75.6662) (34.6243, -69.6759) (37.5374, -68.0703) knots 0 0 0 1 2 2 2
  spline S173 degree 2 poles (37.5374, -68.0703) (40.4649, -66.4567) (45.763, -69.5534) (48.3224, -74.197) knots 0 0 0 1 2 2 2
  spline S174 degree 2 poles (48.2538, -81.3045) (48.115, -80.2341) (46.9091, -77.3639) (45.8996, -75.5324) knots 0 0 0 1 2 2 2
  spline S175 degree 2 poles (45.8996, -75.5324) (44.8902, -73.7009) (43.1153, -71.1631) (42.254, -70.4533) knots 0 0 0 1 2 2 2
  spline S176 degree 2 poles (42.254, -70.4533) (41.3927, -69.7434) (39.6214, -69.4976) (38.6264, -70.046) knots 0 0 0 1 2 2 2
  spline S177 degree 2 poles (38.6264, -70.046) (37.6313, -70.5945) (36.8645, -72.2393) (37.0062, -73.3834) knots 0 0 0 1 2 2 2
  spline S178 degree 2 poles (37.0062, -73.3834) (37.1464, -74.4906) (38.413, -77.4026) (39.3747, -79.1476) knots 0 0 0 1 2 2 2
  spline S179 degree 2 poles (39.3747, -79.1476) (40.4081, -81.0223) (42.0219, -83.4044) (42.9373, -84.1784) knots 0 0 0 1 2 2 2
  spline S180 degree 2 poles (42.9373, -84.1784) (43.7922, -84.9106) (45.6241, -85.1983) (46.6624, -84.626) knots 0 0 0 1 2 2 2
  spline S181 degree 2 poles (46.6624, -84.626) (47.6431, -84.0855) (48.4099, -82.4406) (48.2538, -81.3045) knots 0 0 0 1 2 2 2
  line L200 (64.4848, -74.6062) -> (56.6432, -80.6706)
  line L201 (56.6432, -80.6706) -> (55.3739, -79.0294)
  line L202 (55.3739, -79.0294) -> (58.2917, -76.7729)
  line L203 (58.2917, -76.7729) -> (49.9606, -66.0005)
  line L204 (49.9606, -66.0005) -> (47.0428, -68.257)
  line L205 (47.0428, -68.257) -> (45.9045, -66.7851)
  spline S182 degree 2 poles (45.9045, -66.7851) (47.5588, -65.5057) (48.3966, -63.359) (47.4934, -61.9758) knots 0 0 0 1 2 2 2
  line L206 (47.4934, -61.9758) -> (49.1607, -60.6864)
  line L207 (49.1607, -60.6864) -> (60.3628, -75.1711)
  line L208 (60.3628, -75.1711) -> (63.2155, -72.9649)
  line L209 (63.2155, -72.9649) -> (64.4848, -74.6062)
  spline S183 degree 2 poles (71.8452, -68.0061) (70.8038, -69.1063) (68.4368, -70.2895) (67.2269, -70.346) knots 0 0 0 1 2 2 2
  spline S184 degree 2 poles (67.2269, -70.346) (66.0403, -70.4019) (63.8027, -69.5081) (62.8818, -68.6365) knots 0 0 0 1 2 2 2
  spline S185 degree 2 poles (62.8818, -68.6365) (61.6859, -67.5045) (60.8881, -64.3232) (61.4447, -62.5374) knots 0 0 0 1 2 2 2
  line L210 (61.4447, -62.5374) -> (61.3849, -62.4808)
  spline S186 degree 2 poles (61.3849, -62.4808) (59.721, -62.9691) (57.218, -62.5952) (56.0939, -61.5311) knots 0 0 0 1 2 2 2
  spline S187 degree 2 poles (56.0939, -61.5311) (54.4316, -59.9576) (54.5844, -55.3408) (56.4183, -53.4034) knots 0 0 0 1 2 2 2
  spline S188 degree 2 poles (56.4183, -53.4034) (58.32, -51.3943) (62.7227, -50.959) (64.373, -52.5211) knots 0 0 0 1 2 2 2
  spline S189 degree 2 poles (64.373, -52.5211) (65.3656, -53.4607) (66.2049, -56.4545) (65.7249, -58.0635) knots 0 0 0 1 2 2 2
  line L211 (65.7249, -58.0635) -> (65.7847, -58.1201)
  spline S190 degree 2 poles (65.7847, -58.1201) (67.6052, -57.3945) (70.5838, -57.6971) (71.9471, -58.9876) knots 0 0 0 1 2 2 2
  spline S191 degree 2 poles (71.9471, -58.9876) (73.8366, -60.7761) (73.7923, -65.9491) (71.8452, -68.0061) knots 0 0 0 1 2 2 2
  spline S192 degree 2 poles (70.2141, -61.2017) (69.3052, -60.3414) (67.5497, -60.0402) (66.0374, -60.536) knots 0 0 0 1 2 2 2
  spline S193 degree 2 poles (66.0374, -60.536) (65.5291, -60.6897) (64.0226, -61.395) (63.0677, -61.8289) knots 0 0 0 1 2 2 2
  spline S194 degree 2 poles (63.0677, -61.8289) (62.8361, -63.1515) (63.6122, -65.5413) (64.6287, -66.5035) knots 0 0 0 1 2 2 2
  spline S195 degree 2 poles (64.6287, -66.5035) (65.9681, -67.7714) (69.2423, -67.8096) (70.3969, -66.5898) knots 0 0 0 1 2 2 2
  spline S196 degree 2 poles (70.3969, -66.5898) (71.5742, -65.3461) (71.5056, -62.4243) (70.2141, -61.2017) knots 0 0 0 1 2 2 2
  spline S197 degree 2 poles (62.5631, -54.4811) (61.5705, -53.5416) (58.9866, -53.6125) (57.8659, -54.7964) knots 0 0 0 1 2 2 2
  spline S198 degree 2 poles (57.8659, -54.7964) (56.8471, -55.8727) (56.7293, -58.3687) (57.7458, -59.3308) knots 0 0 0 1 2 2 2
  spline S199 degree 2 poles (57.7458, -59.3308) (58.4753, -60.0214) (60.1597, -60.278) (61.2341, -59.9573) knots 0 0 0 1 2 2 2
  spline S200 degree 2 poles (61.2341, -59.9573) (61.6846, -59.8168) (63.4704, -59.1038) (64.1246, -58.7481) knots 0 0 0 1 2 2 2
  spline S201 degree 2 poles (64.1246, -58.7481) (64.2819, -57.2644) (63.46, -55.3301) (62.5631, -54.4811) knots 0 0 0 1 2 2 2
  constraints: 1 centre point, 1 coincident, 2 other
extrude "Extrusion15" cut sketch "Sketch22" against normal blind 2.54 contours L0 L1 L2 L3 L4 L5 L6 L7 L8 L9 | L10 L11 L12 L13 L14 L15 L16 L17 L18 L19 L20 L21 | S0 S1 S2 S3 S4 S5 L22 L23 S6 S7 S8 S9 S10 S11 S12 S13 L24 L25 S14 S15 | L26 L27 L28 L29 L30 L31 L32 L33 L34 L35 L36 L37 | S16 S17 S18 S19 S20 S21 S22 S23 | L38 L39 L40 L41 L42 L43 | S30 L44 L45 S31 S32 S33 S34 S35 S36 S37 S38 L46 L47 S39 S40 S41 S42 S43 S44 S45 | S46 L48 L49 S47 S48 S49 S50 S51 S52 S53 S54 L50 L51 S55 S56 S57 S58 S59 S60 S61 | S62 S63 S64 S65 S66 S67 L52 L53 S68 S69 S70 S71 S72 S73 S74 S75 L54 L55 S76 S77 | L56 L57 L58 L59 L60 L61 L62 L63 L64 L65 L66 L67 | S78 S79 S80 S81 S82 S83 S84 S85 | S92 S93 S94 S95 S96 S97 S98 S99 | L68 L69 L70 L71 L72 L73 | L74 L75 L76 L77 L78 L79 L80 L81 L82 L83 | L84 L85 L86 L87 L88 L89 L90 S106 S107 S108 L91 | S113 S114 S115 S116 S117 S118 L95 L96 S119 S120 S121 S122 S123 S124 S125 S126 L97 L98 S127 S128 | S129 S130 L99 L100 L101 L102 L103 S131 S132 | L107 L108 L119 L109 L110 L111 L112 L113 L114 L115 L116 L117 L118 | L119 L120 L137 L136 L122 L123 L124 L125 L126 L127 L128 L129 L130 L109 L108 | L108 L109 L119 | L137 S137 S138 S139 L138 L131 L132 L133 L134 L135 L136 L122 L121 L120 | L120 L121 L122 L136 L137 | L142 L143 L144 L145 L146 L147 L148 L149 | L153 L154 L155 L156 L157 L158 L159 L160 L161 L162 L163 L164 L165 | L166 L167 L168 L169 L170 L171 L172 L173 | L177 L178 L179 L180 L181 L182 L183 S144 S145 S146 L184 | S151 S152 L188 L189 L190 S153 S154 | L194 L195 S159 S160 S161 S162 S163 S164 L196 L197 S165 S166 S167 S168 S169 L198 L199 | S170 S171 S172 S173 | L200 L201 L202 L203 L204 L205 S182 L206 L207 L208 L209 | S183 S184 S185 L210 S186 S187 S188 S189 L211 S190 S191
sketch "Sketch23" plane through (0, 0, 0) normal (-1, 0, 0) x (0, 0, 1)
  point P0 (0, 0)
sketch "Sketch24" plane through (0, 0, 0) normal (-1, 0, 0) x (0, 0, 1)
  point P0 (0, 0)